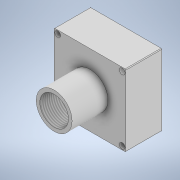
# Autodesk Inventor part: Tarea 1 Joel Monroy Lab Din
Saved by Autodesk Inventor 2021 (Build 250183000, 183)
## iProperties
Created: 2024-02-06
Part Number: Tarea 1 Joel Monroy Lab Din
Material: Genérico
Document SubType Name: Modeling
Designer: joelm
Density: 1 g/cm^3
Appearance: Valor por defecto
Author: joelm
Autodesk Inventor part; units mm, degrees
ref_plane "YZ Plane" through (0, 0, 0) normal (1, 0, 0) x (0, 1, 0)
ref_plane "XZ Plane" through (0, 0, 0) normal (0, 1, 0) x (-1, 0, 0)
ref_plane "XY Plane" through (0, 0, 0) normal (0, 0, 1) x (1, 0, 0)
sketch "Boceto1" plane through (0, 0, 0) normal (0, 0, 1) x (1, 0, 0)
  line L0 (0, 0) -> (100, 0)
  line L1 (100, 0) -> (100, 100)
  line L2 (100, 100) -> (0, 100)
  line L3 (0, 100) -> (0, 0)
  line L4 (0, 100) -> (5, 100)
  circle A0 centre (5, 95) radius 4
  line L5 (0, 0) -> (0, 5)
  circle A1 centre (5, 5) radius 4
  line L6 (100, 0) -> (100, 5)
  circle A2 centre (95, 5) radius 4
  line L7 (100, 100) -> (95, 100)
  circle A3 centre (95, 95) radius 4
  line L8 (0, 100) -> (50, 100)
  line L9 (50, 100) -> (50, 50)
  dimension "d6" = 100
  dimension "d7" = 100
  dimension "d10" = 8
  dimension "d20" = 50
  dimension "d21" = 50
  constraints: 20 end point, 4 centre point, 4 point on line, 2 parallel, 2 perpendicular, 1 horizontal, 1 midpoint
  measures "d6" distance of L2.end L1.end
  measures "d7" distance of L1.end L0.end
  measures "d10" diameter of A0
  measures "d20" distance of L2.end L8.end
  measures "d21" distance of L8.end L9.end
extrude "Extrusión1" add sketch "Boceto1" along normal blind 50
fillet "Empalme1" radius 1 4 edges at (100, 0, 25) (0, 0, 25) (100, 100, 25) (0, 100, 25)
sketch "Boceto2" plane through (0, 0, 50) normal (0, 0, 1) x (1, 0, 0)
  circle A0 centre (50, 50) radius 25
  point P0 (0, 0)
  dimension "d27" = 50
  constraints: 1 centre point
  measures "d27" diameter of A0
extrude "Extrusión2" add sketch "Boceto2" along normal blind 50
sketch "Boceto3" plane through (50, 50, 100) normal (0, 0, 1) x (1, 0, 0)
  circle A0 centre (0, 0) radius 20
  point P0 (-50, -50)
  dimension "d30" = 40
  constraints: 1 centre point
  measures "d30" diameter of A0
extrude "Extrusión3" cut sketch "Boceto3" against normal blind 30
thread "Rosca1" size "M40x3" class "6H" standard "ANSI Metric M Profile" length 30
